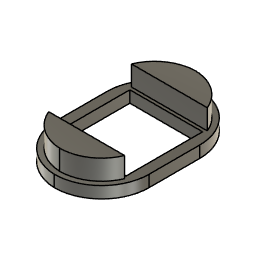
ballzfretstabilizer (Autodesk Fusion 360 design; units mm, degrees)
Autodesk Fusion 360 part; units mm, degrees
note: some values were not read from the file. Set by a fixed rule: which sketch regions a step uses.
sketch "Sketch1" plane through (0, 0, 0) normal (0, 0, 1) x (1, 0, 0)
  line L0 (8.8, -8.8) -> (-8.8, -8.8)
  line L1 (-8.8, -8.8) -> (-8.8, 8.8)
  line L2 (-8.8, 8.8) -> (8.8, 8.8)
  line L3 (8.8, 8.8) -> (8.8, -8.8)
  line L4 (8.8, -8.8) -> (-8.8, 8.8) construction
  line L5 (-8.8, -8.8) -> (8.8, 8.8) construction
  dimension "d1" = 17.6
  dimension "d2" = 17.6
  constraint horizontal L0
  constraint perpendicular L0 L1
  constraint parallel L0 L2
  constraint parallel L1 L3
  constraint coincident L4 origin
  constraint coincident L5 origin
  measures "d1" distance of L1.end L2.end
  measures "d2" distance of L0.end L1.end
extrude "Extrude1" add sketch "Sketch1" along normal blind 2.2
sketch "Sketch2" plane through (0, 0, 2.2) normal (0, 0, 1) x (-1, 0, 0)
  line L0 (-8.8, -8.8) -> (8.8, -8.8)
  line L1 (8.8, -8.8) -> (8.8, 8.8)
  line L2 (8.8, 8.8) -> (-8.8, 8.8)
  line L3 (-8.8, 8.8) -> (-8.8, -8.8)
  line L4 (6.9, 7.25) -> (-6.9, 7.25)
  line L5 (-6.9, 7.25) -> (-6.9, -7.25)
  line L6 (-6.9, -7.25) -> (6.9, -7.25)
  line L7 (6.9, -7.25) -> (6.9, 7.25)
  line L8 (6.9, 7.25) -> (-6.9, -7.25) construction
  line L9 (-6.9, 7.25) -> (6.9, -7.25) construction
  dimension "d5" = 13.8
  dimension "d6" = 14.5
  constraint horizontal L4
  constraint perpendicular L4 L5
  constraint parallel L4 L6
  constraint parallel L5 L7
  constraint coincident L8 origin
  constraint coincident L9 origin
  measures "d5" distance of L5.end L6.end
  measures "d6" distance of L4.end L5.end
extrude "Extrude2" cut sketch "Sketch2" against normal blind 2.2 contours L4 L5 L6 L7
extrude "Extrude3" add 1 faces at (2.9333, -8.8, 1.4667) along direction (0, -1, 0) blind 5
extrude "Extrude4" add 1 faces at (-2.9333, 8.8, 1.4667) along direction (0, 1, 0) blind 5
fillet "Fillet1" radius 9 2 edges at (8.8, 13.8, 1.1) (-8.8, 13.8, 1.1)
fillet "Fillet2" radius 9 2 edges at (8.8, -13.8, 1.1) (-8.8, -13.8, 1.1)
sketch "Sketch4" plane through (0, 0, 2.2) normal (0, 0, 1) x (-1, 0, 0)
  arc A0 (8.8, 4.8089) -> (0.2, 13.8) centre (-0.2, 4.8089) ccw
  arc A1 (0.2, 13.8) -> (-8.8, 4.8) centre (0.2, 4.8) ccw
  line L0 (-8.8, 4.8) -> (-8.8, -4.8)
  arc A2 (-8.8, -4.8) -> (0.2, -13.8) centre (0.2, -4.8) ccw
  arc A3 (0.2, -13.8) -> (8.8, -4.8089) centre (-0.2, -4.8089) ccw
  line L1 (8.8, -4.8089) -> (8.8, 4.8089)
  line L2 (-6.9, 7.25) -> (6.9, 7.25)
  line L3 (6.9, 7.25) -> (6.9, -7.25)
  line L4 (6.9, -7.25) -> (-6.9, -7.25)
  line L5 (-6.9, -7.25) -> (-6.9, 7.25)
  line L6 (0, 7.25) -> (0, 7.85)
  line L7 (0, -7.25) -> (0, -7.85)
  line L8 (-7.8, 7.85) -> (7.8, 7.85)
  line L9 (-7.1958, -7.85) -> (7.1994, -7.85)
  line L10 (-7.8, 4.8) -> (-7.8, -4.8)
  arc A4 (-7.8, -4.8) -> (0.1778, -12.8) centre (0.2, -4.8) ccw
  arc A5 (0.1778, -12.8) -> (7.8, -4.8089) centre (-0.2, -4.8089) ccw
  line L11 (7.8, -4.8089) -> (7.8, 4.8089)
  arc A6 (7.8, 4.8089) -> (0.1778, 12.8) centre (-0.2, 4.8089) ccw
  arc A7 (0.1778, 12.8) -> (-7.8, 4.8) centre (0.2, 4.8) ccw
  dimension "d18" = -1
  dimension "d19" = 0.6
  dimension "d20" = 0.6
  constraint midpoint L2 L6.start
  constraint perpendicular L2 L6
  constraint midpoint L4 L7.start
  constraint perpendicular L4 L7
  constraint coincident L8.start L10
  constraint coincident L8.end L11
  constraint perpendicular L8 L11
  constraint coincident L9.start A4
  constraint coincident L9.end A5
  constraint perpendicular L7 L9
  measures "d19" distance of L6.start L6.end
  measures "d20" distance of L7.start L7.end
extrude "Extrude5" add sketch "Sketch4" along normal blind 3.8 contours L8 A6 A7 | L9 A4 A5
